Autodesk Fusion 360 part; units mm, degrees
(part 2 of 2)
  spline S13 degree 5 poles (-231.6326, -210.6007) (-231.5801, -210.5749) (-231.4751, -210.5231) (-231.318, -210.4449) (-231.1091, -210.34) (-230.8492, -210.2076) (-230.5904, -210.0739) (-230.3328, -209.9389) (-230.0763, -209.8027) (-229.821, -209.6652) (-229.5668, -209.5264) (-229.3139, -209.3863) (-229.0621, -209.245) (-228.8116, -209.1023) (-228.5623, -208.9584) (-228.3143, -208.8132) (-228.0675, -208.6668) (-227.8221, -208.5191) (-227.5779, -208.37) (-227.335, -208.2197) (-227.0934, -208.0681) (-226.8532, -207.9153) (-226.6143, -207.7611) (-226.3769, -207.6057) (-226.1408, -207.4489) (-225.9061, -207.2909) (-225.6728, -207.1316) (-225.4409, -206.971) (-225.2106, -206.8091) (-224.9817, -206.6459) (-224.7543, -206.4813) (-224.5284, -206.3155) (-224.304, -206.1484) (-224.0813, -205.9799) (-223.8601, -205.8102) (-223.6405, -205.6391) (-223.4226, -205.4667) (-223.2062, -205.2929) (-222.9916, -205.1179) (-222.7786, -204.9415) (-222.5674, -204.7638) (-222.358, -204.5847) (-222.1504, -204.4042) (-221.9447, -204.2224) (-221.7408, -204.0391) (-221.5388, -203.8546) (-221.3387, -203.6686) (-221.1405, -203.4813) (-220.9443, -203.2926) (-220.75, -203.1025) (-220.5579, -202.911) (-220.368, -202.718) (-220.1805, -202.5234) (-219.9954, -202.3273) (-219.8127, -202.1296) (-219.6323, -201.9304) (-219.4541, -201.7299) (-219.278, -201.528) (-219.104, -201.3248) (-218.9326, -201.12) (-218.7643, -200.9135) (-218.5996, -200.7049) (-218.4389, -200.494) (-218.2823, -200.2809) (-218.1292, -200.0659) (-217.979, -199.8493) (-217.8307, -199.6317) (-217.6843, -199.4131) (-217.5406, -199.1931) (-217.4019, -198.9707) (-217.2716, -198.7443) (-217.1767, -198.5586) (-217.112, -198.4162) (-217.0719, -198.3197) (-217.0526, -198.2711) knots -1 -1 -1 -1 -1 -1 -0.98571429 -0.97142857 -0.95714286 -0.94285714 -0.92857143 -0.91428571 -0.9 -0.88571429 -0.87142857 -0.85714286 -0.84285714 -0.82857143 -0.81428571 -0.8 -0.78571429 -0.77142857 -0.75714286 -0.74285714 -0.72857143 -0.71428571 -0.7 -0.68571429 -0.67142857 -0.65714286 -0.64285714 -0.62857143 -0.61428571 -0.6 -0.58571429 -0.57142857 -0.55714286 -0.54285714 -0.52857143 -0.51428571 -0.5 -0.48571429 -0.47142857 -0.45714286 -0.44285714 -0.42857143 -0.41428571 -0.4 -0.38571429 -0.37142857 -0.35714286 -0.34285714 -0.32857143 -0.31428571 -0.3 -0.28571429 -0.27142857 -0.25714286 -0.24285714 -0.22857143 -0.21428571 -0.2 -0.18571429 -0.17142857 -0.15714286 -0.14285714 -0.12857143 -0.11428571 -0.1 -0.08571429 -0.07142857 -0.05714286 -0.04285714 -0.02857143 -0.01428571 0 0 0 0 0 0
  line L13 (-217.0526, -198.2711) -> (-214.0537, -190.7145)
  arc A27 (-211.5159, -189.5709) -> (-214.0537, -190.7145) centre (-212.1947, -191.4522) ccw
  arc A28 (-211.5159, -189.5709) -> (-201.4878, -192.2579) centre (-190.6397, -131.7161) ccw
  arc A29 (-199.8618, -194.5172) -> (-201.4878, -192.2579) centre (-201.8406, -194.2266) ccw
  line L14 (-199.8618, -194.5172) -> (-201.043, -202.5609)
  spline S14 degree 5 poles (-201.043, -202.5609) (-201.0506, -202.6126) (-201.0641, -202.7162) (-201.0793, -202.8719) (-201.09, -203.0801) (-201.0903, -203.3414) (-201.0814, -203.6034) (-201.0669, -203.8657) (-201.0494, -204.1282) (-201.0299, -204.3908) (-201.008, -204.6535) (-200.983, -204.9163) (-200.9539, -205.1791) (-200.9201, -205.4421) (-200.8818, -205.7051) (-200.8393, -205.9681) (-200.7932, -206.2312) (-200.7443, -206.4941) (-200.6927, -206.757) (-200.6386, -207.0198) (-200.5819, -207.2825) (-200.5225, -207.545) (-200.4603, -207.8074) (-200.3952, -208.0696) (-200.3273, -208.3318) (-200.2567, -208.5937) (-200.1835, -208.8554) (-200.1078, -209.117) (-200.0298, -209.3783) (-199.9495, -209.6394) (-199.8669, -209.9002) (-199.782, -210.1609) (-199.6947, -210.4212) (-199.6052, -210.6813) (-199.5133, -210.9411) (-199.4193, -211.2006) (-199.3231, -211.4598) (-199.2247, -211.7188) (-199.1242, -211.9774) (-199.0217, -212.2357) (-198.9171, -212.4936) (-198.8104, -212.7512) (-198.7017, -213.0085) (-198.591, -213.2654) (-198.4783, -213.522) (-198.3636, -213.7781) (-198.247, -214.0339) (-198.1284, -214.2893) (-198.008, -214.5444) (-197.8856, -214.799) (-197.7613, -215.0532) (-197.6352, -215.307) (-197.5073, -215.5603) (-197.3775, -215.8133) (-197.2459, -216.0658) (-197.1125, -216.3178) (-196.9773, -216.5694) (-196.8403, -216.8206) (-196.7016, -217.0713) (-196.5611, -217.3215) (-196.4189, -217.5712) (-196.275, -217.8205) (-196.1294, -218.0693) (-195.982, -218.3175) (-195.833, -218.5653) (-195.6823, -218.8126) (-195.53, -219.0593) (-195.376, -219.3056) (-195.2203, -219.5513) (-195.063, -219.7965) (-194.9042, -220.0411) (-194.7758, -220.2364) (-194.6787, -220.3826) (-194.6137, -220.48) (-194.5811, -220.5287) knots 0 0 0 0 0 0 0.01428571 0.02857143 0.04285714 0.05714286 0.07142857 0.08571429 0.1 0.11428571 0.12857143 0.14285714 0.15714286 0.17142857 0.18571429 0.2 0.21428571 0.22857143 0.24285714 0.25714286 0.27142857 0.28571429 0.3 0.31428571 0.32857143 0.34285714 0.35714286 0.37142857 0.38571429 0.4 0.41428571 0.42857143 0.44285714 0.45714286 0.47142857 0.48571429 0.5 0.51428571 0.52857143 0.54285714 0.55714286 0.57142857 0.58571429 0.6 0.61428571 0.62857143 0.64285714 0.65714286 0.67142857 0.68571429 0.7 0.71428571 0.72857143 0.74285714 0.75714286 0.77142857 0.78571429 0.8 0.81428571 0.82857143 0.84285714 0.85714286 0.87142857 0.88571429 0.9 0.91428571 0.92857143 0.94285714 0.95714286 0.97142857 0.98571429 1 1 1 1 1 1
  arc A30 (-194.5811, -220.5287) -> (-186.6983, -220.5287) centre (-190.6397, -131.7161) ccw
  spline S15 degree 5 poles (-186.6983, -220.5287) (-186.6657, -220.48) (-186.6007, -220.3826) (-186.5037, -220.2364) (-186.3753, -220.0411) (-186.2164, -219.7965) (-186.0591, -219.5513) (-185.9035, -219.3056) (-185.7495, -219.0593) (-185.5971, -218.8126) (-185.4464, -218.5653) (-185.2974, -218.3175) (-185.1501, -218.0693) (-185.0044, -217.8205) (-184.8605, -217.5712) (-184.7183, -217.3215) (-184.5778, -217.0713) (-184.4391, -216.8206) (-184.3021, -216.5694) (-184.1669, -216.3178) (-184.0335, -216.0658) (-183.9019, -215.8133) (-183.7721, -215.5603) (-183.6442, -215.307) (-183.5181, -215.0532) (-183.3938, -214.799) (-183.2715, -214.5444) (-183.151, -214.2893) (-183.0324, -214.0339) (-182.9158, -213.7781) (-182.8011, -213.522) (-182.6884, -213.2654) (-182.5777, -213.0085) (-182.469, -212.7512) (-182.3624, -212.4936) (-182.2577, -212.2357) (-182.1552, -211.9774) (-182.0547, -211.7188) (-181.9564, -211.4598) (-181.8601, -211.2006) (-181.7661, -210.9411) (-181.6743, -210.6813) (-181.5847, -210.4212) (-181.4975, -210.1609) (-181.4125, -209.9002) (-181.3299, -209.6394) (-181.2496, -209.3783) (-181.1716, -209.117) (-181.096, -208.8554) (-181.0228, -208.5937) (-180.9521, -208.3318) (-180.8842, -208.0696) (-180.8191, -207.8074) (-180.7569, -207.545) (-180.6975, -207.2825) (-180.6409, -207.0198) (-180.5868, -206.757) (-180.5352, -206.4941) (-180.4862, -206.2312) (-180.4401, -205.9681) (-180.3976, -205.7051) (-180.3593, -205.4421) (-180.3255, -205.1791) (-180.2964, -204.9163) (-180.2714, -204.6535) (-180.2496, -204.3908) (-180.23, -204.1282) (-180.2125, -203.8657) (-180.1981, -203.6034) (-180.1891, -203.3414) (-180.1895, -203.0801) (-180.2001, -202.8719) (-180.2153, -202.7162) (-180.2288, -202.6126) (-180.2364, -202.5609) knots -1 -1 -1 -1 -1 -1 -0.98571429 -0.97142857 -0.95714286 -0.94285714 -0.92857143 -0.91428571 -0.9 -0.88571429 -0.87142857 -0.85714286 -0.84285714 -0.82857143 -0.81428571 -0.8 -0.78571429 -0.77142857 -0.75714286 -0.74285714 -0.72857143 -0.71428571 -0.7 -0.68571429 -0.67142857 -0.65714286 -0.64285714 -0.62857143 -0.61428571 -0.6 -0.58571429 -0.57142857 -0.55714286 -0.54285714 -0.52857143 -0.51428571 -0.5 -0.48571429 -0.47142857 -0.45714286 -0.44285714 -0.42857143 -0.41428571 -0.4 -0.38571429 -0.37142857 -0.35714286 -0.34285714 -0.32857143 -0.31428571 -0.3 -0.28571429 -0.27142857 -0.25714286 -0.24285714 -0.22857143 -0.21428571 -0.2 -0.18571429 -0.17142857 -0.15714286 -0.14285714 -0.12857143 -0.11428571 -0.1 -0.08571429 -0.07142857 -0.05714286 -0.04285714 -0.02857143 -0.01428571 0 0 0 0 0 0
  line L15 (-180.2364, -202.5609) -> (-181.4176, -194.5172)
  arc A31 (-179.7916, -192.2579) -> (-181.4176, -194.5172) centre (-179.4388, -194.2266) ccw
  arc A32 (-179.7916, -192.2579) -> (-169.7635, -189.5709) centre (-190.6397, -131.7161) ccw
  arc A33 (-167.2257, -190.7145) -> (-169.7635, -189.5709) centre (-169.0847, -191.4522) ccw
  line L16 (-167.2257, -190.7145) -> (-164.2268, -198.2711)
  spline S16 degree 5 poles (-164.2268, -198.2711) (-164.2075, -198.3197) (-164.1675, -198.4162) (-164.1028, -198.5586) (-164.0079, -198.7443) (-163.8775, -198.9707) (-163.7388, -199.1931) (-163.5951, -199.4131) (-163.4487, -199.6317) (-163.3005, -199.8493) (-163.1502, -200.0659) (-162.9972, -200.2809) (-162.8405, -200.494) (-162.6798, -200.7049) (-162.5151, -200.9135) (-162.3468, -201.12) (-162.1754, -201.3248) (-162.0015, -201.528) (-161.8253, -201.7299) (-161.6471, -201.9304) (-161.4667, -202.1296) (-161.284, -202.3273) (-161.099, -202.5234) (-160.9114, -202.718) (-160.7216, -202.911) (-160.5294, -203.1025) (-160.3352, -203.2926) (-160.1389, -203.4813) (-159.9407, -203.6686) (-159.7406, -203.8546) (-159.5386, -204.0391) (-159.3348, -204.2224) (-159.129, -204.4042) (-158.9214, -204.5847) (-158.712, -204.7638) (-158.5008, -204.9415) (-158.2878, -205.1179) (-158.0732, -205.2929) (-157.8569, -205.4667) (-157.6389, -205.6391) (-157.4193, -205.8102) (-157.1982, -205.9799) (-156.9754, -206.1484) (-156.7511, -206.3155) (-156.5252, -206.4813) (-156.2978, -206.6459) (-156.0689, -206.8091) (-155.8385, -206.971) (-155.6067, -207.1316) (-155.3734, -207.2909) (-155.1387, -207.4489) (-154.9026, -207.6057) (-154.6651, -207.7611) (-154.4262, -207.9153) (-154.186, -208.0681) (-153.9444, -208.2197) (-153.7016, -208.37) (-153.4574, -208.5191) (-153.2119, -208.6668) (-152.9651, -208.8132) (-152.7171, -208.9584) (-152.4678, -209.1023) (-152.2173, -209.245) (-151.9656, -209.3863) (-151.7126, -209.5264) (-151.4585, -209.6652) (-151.2031, -209.8027) (-150.9467, -209.9389) (-150.689, -210.0739) (-150.4302, -210.2076) (-150.1703, -210.34) (-149.9615, -210.4449) (-149.8043, -210.5231) (-149.6993, -210.5749) (-149.6468, -210.6007) knots 0 0 0 0 0 0 0.01428571 0.02857143 0.04285714 0.05714286 0.07142857 0.08571429 0.1 0.11428571 0.12857143 0.14285714 0.15714286 0.17142857 0.18571429 0.2 0.21428571 0.22857143 0.24285714 0.25714286 0.27142857 0.28571429 0.3 0.31428571 0.32857143 0.34285714 0.35714286 0.37142857 0.38571429 0.4 0.41428571 0.42857143 0.44285714 0.45714286 0.47142857 0.48571429 0.5 0.51428571 0.52857143 0.54285714 0.55714286 0.57142857 0.58571429 0.6 0.61428571 0.62857143 0.64285714 0.65714286 0.67142857 0.68571429 0.7 0.71428571 0.72857143 0.74285714 0.75714286 0.77142857 0.78571429 0.8 0.81428571 0.82857143 0.84285714 0.85714286 0.87142857 0.88571429 0.9 0.91428571 0.92857143 0.94285714 0.95714286 0.97142857 0.98571429 1 1 1 1 1 1
  arc A34 (-149.6468, -210.6007) -> (-142.8201, -206.6593) centre (-190.6397, -131.7161) ccw
  spline S17 degree 5 poles (-142.8201, -206.6593) (-142.8162, -206.6009) (-142.8086, -206.484) (-142.7976, -206.3089) (-142.7841, -206.0756) (-142.7688, -205.7843) (-142.7552, -205.4933) (-142.7433, -205.2027) (-142.733, -204.9124) (-142.7244, -204.6226) (-142.7176, -204.3331) (-142.7124, -204.044) (-142.7089, -203.7553) (-142.7072, -203.467) (-142.7072, -203.1792) (-142.7089, -202.8918) (-142.7124, -202.6049) (-142.7176, -202.3184) (-142.7245, -202.0324) (-142.7332, -201.7469) (-142.7437, -201.462) (-142.756, -201.1775) (-142.7701, -200.8935) (-142.786, -200.6101) (-142.8036, -200.3273) (-142.8232, -200.045) (-142.8445, -199.7633) (-142.8677, -199.4823) (-142.8927, -199.2018) (-142.9196, -198.922) (-142.9484, -198.6428) (-142.979, -198.3642) (-143.0116, -198.0864) (-143.0461, -197.8092) (-143.0825, -197.5328) (-143.1209, -197.2571) (-143.1612, -196.9821) (-143.2035, -196.7079) (-143.2478, -196.4345) (-143.2941, -196.1619) (-143.3424, -195.8901) (-143.3928, -195.6192) (-143.4453, -195.3492) (-143.4999, -195.0801) (-143.5566, -194.812) (-143.6155, -194.5447) (-143.6765, -194.2785) (-143.7396, -194.0132) (-143.8049, -193.7488) (-143.8724, -193.4856) (-143.9422, -193.2234) (-144.0144, -192.9625) (-144.0892, -192.7028) (-144.1665, -192.4444) (-144.2463, -192.1874) (-144.3286, -191.9316) (-144.4131, -191.677) (-144.4999, -191.4235) (-144.589, -191.1713) (-144.6806, -190.9204) (-144.7753, -190.6714) (-144.8736, -190.4244) (-144.9759, -190.1798) (-145.0821, -189.9377) (-145.1918, -189.6976) (-145.3042, -189.4592) (-145.4186, -189.222) (-145.5347, -188.9859) (-145.6533, -188.7515) (-145.7766, -188.5202) (-145.9075, -188.2941) (-146.0209, -188.119) (-146.1119, -187.9918) (-146.1754, -187.9088) (-146.2078, -187.8678) knots -1 -1 -1 -1 -1 -1 -0.98571429 -0.97142857 -0.95714286 -0.94285714 -0.92857143 -0.91428571 -0.9 -0.88571429 -0.87142857 -0.85714286 -0.84285714 -0.82857143 -0.81428571 -0.8 -0.78571429 -0.77142857 -0.75714286 -0.74285714 -0.72857143 -0.71428571 -0.7 -0.68571429 -0.67142857 -0.65714286 -0.64285714 -0.62857143 -0.61428571 -0.6 -0.58571429 -0.57142857 -0.55714286 -0.54285714 -0.52857143 -0.51428571 -0.5 -0.48571429 -0.47142857 -0.45714286 -0.44285714 -0.42857143 -0.41428571 -0.4 -0.38571429 -0.37142857 -0.35714286 -0.34285714 -0.32857143 -0.31428571 -0.3 -0.28571429 -0.27142857 -0.25714286 -0.24285714 -0.22857143 -0.21428571 -0.2 -0.18571429 -0.17142857 -0.15714286 -0.14285714 -0.12857143 -0.11428571 -0.1 -0.08571429 -0.07142857 -0.05714286 -0.04285714 -0.02857143 -0.01428571 0 0 0 0 0 0
  line L17 (-146.2078, -187.8678) -> (-151.2526, -181.4924)
  arc A35 (-150.974, -178.7228) -> (-151.2526, -181.4924) centre (-149.6842, -180.2513) ccw
  arc A36 (-150.974, -178.7228) -> (-143.633, -171.3818) centre (-190.6397, -131.7161) ccw
  arc A37 (-140.8634, -171.1032) -> (-143.633, -171.3818) centre (-142.1045, -172.6716) ccw
  line L18 (-140.8634, -171.1032) -> (-134.488, -176.148)
  spline S18 degree 5 poles (-134.488, -176.148) (-134.447, -176.1804) (-134.364, -176.2439) (-134.2368, -176.3349) (-134.0617, -176.4483) (-133.8356, -176.5792) (-133.6043, -176.7024) (-133.3699, -176.8211) (-133.1338, -176.9372) (-132.8966, -177.0516) (-132.6582, -177.164) (-132.4181, -177.2737) (-132.1759, -177.3799) (-131.9313, -177.4822) (-131.6844, -177.5805) (-131.4353, -177.6752) (-131.1845, -177.7668) (-130.9323, -177.8559) (-130.6788, -177.9427) (-130.4242, -178.0272) (-130.1684, -178.1095) (-129.9114, -178.1893) (-129.653, -178.2666) (-129.3933, -178.3414) (-129.1324, -178.4136) (-128.8702, -178.4834) (-128.6069, -178.5509) (-128.3426, -178.6161) (-128.0773, -178.6793) (-127.811, -178.7403) (-127.5438, -178.7991) (-127.2757, -178.8559) (-127.0066, -178.9105) (-126.7366, -178.963) (-126.4656, -179.0134) (-126.1939, -179.0617) (-125.9213, -179.108) (-125.6478, -179.1522) (-125.3736, -179.1945) (-125.0987, -179.2349) (-124.823, -179.2732) (-124.5466, -179.3097) (-124.2694, -179.3442) (-123.9916, -179.3768) (-123.713, -179.4074) (-123.4338, -179.4362) (-123.154, -179.4631) (-122.8735, -179.4881) (-122.5924, -179.5113) (-122.3108, -179.5326) (-122.0285, -179.5521) (-121.7456, -179.5698) (-121.4622, -179.5857) (-121.1783, -179.5998) (-120.8938, -179.6121) (-120.6088, -179.6225) (-120.3233, -179.6313) (-120.0374, -179.6382) (-119.7509, -179.6434) (-119.464, -179.6469) (-119.1766, -179.6486) (-118.8888, -179.6486) (-118.6005, -179.6468) (-118.3118, -179.6434) (-118.0227, -179.6382) (-117.7332, -179.6313) (-117.4433, -179.6228) (-117.1531, -179.6125) (-116.8625, -179.6006) (-116.5715, -179.587) (-116.2802, -179.5717) (-116.0469, -179.5581) (-115.8717, -179.5472) (-115.7549, -179.5396) (-115.6965, -179.5357) knots 0 0 0 0 0 0 0.01428571 0.02857143 0.04285714 0.05714286 0.07142857 0.08571429 0.1 0.11428571 0.12857143 0.14285714 0.15714286 0.17142857 0.18571429 0.2 0.21428571 0.22857143 0.24285714 0.25714286 0.27142857 0.28571429 0.3 0.31428571 0.32857143 0.34285714 0.35714286 0.37142857 0.38571429 0.4 0.41428571 0.42857143 0.44285714 0.45714286 0.47142857 0.48571429 0.5 0.51428571 0.52857143 0.54285714 0.55714286 0.57142857 0.58571429 0.6 0.61428571 0.62857143 0.64285714 0.65714286 0.67142857 0.68571429 0.7 0.71428571 0.72857143 0.74285714 0.75714286 0.77142857 0.78571429 0.8 0.81428571 0.82857143 0.84285714 0.85714286 0.87142857 0.88571429 0.9 0.91428571 0.92857143 0.94285714 0.95714286 0.97142857 0.98571429 1 1 1 1 1 1
  arc A38 (-115.6965, -179.5357) -> (-111.7551, -172.709) centre (-190.6397, -131.7161) ccw
  spline S19 degree 5 poles (-111.7551, -172.709) (-111.7809, -172.6564) (-111.8327, -172.5515) (-111.9109, -172.3943) (-112.0158, -172.1855) (-112.1482, -171.9255) (-112.2819, -171.6668) (-112.4169, -171.4091) (-112.5531, -171.1526) (-112.6906, -170.8973) (-112.8294, -170.6432) (-112.9695, -170.3902) (-113.1108, -170.1385) (-113.2535, -169.888) (-113.3974, -169.6387) (-113.5425, -169.3907) (-113.689, -169.1439) (-113.8367, -168.8984) (-113.9857, -168.6542) (-114.1361, -168.4113) (-114.2876, -168.1698) (-114.4405, -167.9296) (-114.5947, -167.6907) (-114.7501, -167.4532) (-114.9068, -167.2171) (-115.0649, -166.9824) (-115.2242, -166.7491) (-115.3848, -166.5173) (-115.5467, -166.2869) (-115.7099, -166.058) (-115.8744, -165.8306) (-116.0403, -165.6047) (-116.2074, -165.3804) (-116.3759, -165.1576) (-116.5456, -164.9364) (-116.7167, -164.7169) (-116.8891, -164.4989) (-117.0628, -164.2826) (-117.2379, -164.068) (-117.4143, -163.855) (-117.592, -163.6438) (-117.7711, -163.4344) (-117.9516, -163.2268) (-118.1334, -163.021) (-118.3166, -162.8172) (-118.5012, -162.6152) (-118.6872, -162.4151) (-118.8745, -162.2169) (-119.0632, -162.0206) (-119.2533, -161.8264) (-119.4448, -161.6342) (-119.6378, -161.4443) (-119.8324, -161.2568) (-120.0285, -161.0717) (-120.2262, -160.8891) (-120.4253, -160.7087) (-120.6259, -160.5304) (-120.8277, -160.3543) (-121.031, -160.1804) (-121.2358, -160.009) (-121.4423, -159.8407) (-121.6509, -159.676) (-121.8618, -159.5152) (-122.0748, -159.3586) (-122.2899, -159.2056) (-122.5064, -159.0553) (-122.7241, -158.9071) (-122.9427, -158.7607) (-123.1627, -158.617) (-123.3851, -158.4783) (-123.6115, -158.3479) (-123.7972, -158.253) (-123.9396, -158.1883) (-124.0361, -158.1482) (-124.0847, -158.129) knots -1 -1 -1 -1 -1 -1 -0.98571429 -0.97142857 -0.95714286 -0.94285714 -0.92857143 -0.91428571 -0.9 -0.88571429 -0.87142857 -0.85714286 -0.84285714 -0.82857143 -0.81428571 -0.8 -0.78571429 -0.77142857 -0.75714286 -0.74285714 -0.72857143 -0.71428571 -0.7 -0.68571429 -0.67142857 -0.65714286 -0.64285714 -0.62857143 -0.61428571 -0.6 -0.58571429 -0.57142857 -0.55714286 -0.54285714 -0.52857143 -0.51428571 -0.5 -0.48571429 -0.47142857 -0.45714286 -0.44285714 -0.42857143 -0.41428571 -0.4 -0.38571429 -0.37142857 -0.35714286 -0.34285714 -0.32857143 -0.31428571 -0.3 -0.28571429 -0.27142857 -0.25714286 -0.24285714 -0.22857143 -0.21428571 -0.2 -0.18571429 -0.17142857 -0.15714286 -0.14285714 -0.12857143 -0.11428571 -0.1 -0.08571429 -0.07142857 -0.05714286 -0.04285714 -0.02857143 -0.01428571 0 0 0 0 0 0
  line L19 (-124.0847, -158.129) -> (-131.6413, -155.13)
  arc A39 (-132.7849, -152.5923) -> (-131.6413, -155.13) centre (-130.9036, -153.2711) ccw
  arc A40 (-132.7849, -152.5923) -> (-130.0978, -142.5642) centre (-190.6397, -131.7161) ccw
  arc A41 (-127.8386, -140.9382) -> (-130.0978, -142.5642) centre (-128.1292, -142.9169) ccw
  line L20 (-127.8386, -140.9382) -> (-119.7949, -142.1194)
  spline S20 degree 5 poles (-119.7949, -142.1194) (-119.7432, -142.127) (-119.6396, -142.1405) (-119.4839, -142.1557) (-119.2756, -142.1663) (-119.0144, -142.1666) (-118.7524, -142.1577) (-118.4901, -142.1432) (-118.2276, -142.1258) (-117.9649, -142.1062) (-117.7023, -142.0844) (-117.4395, -142.0594) (-117.1767, -142.0303) (-116.9137, -141.9965) (-116.6507, -141.9581) (-116.3877, -141.9156) (-116.1246, -141.8696) (-115.8616, -141.8206) (-115.5988, -141.769) (-115.336, -141.7149) (-115.0733, -141.6583) (-114.8108, -141.5989) (-114.5484, -141.5367) (-114.2861, -141.4716) (-114.024, -141.4036) (-113.7621, -141.333) (-113.5004, -141.2598) (-113.2388, -141.1842) (-112.9775, -141.1062) (-112.7164, -141.0259) (-112.4555, -140.9433) (-112.1949, -140.8583) (-111.9346, -140.7711) (-111.6745, -140.6815) (-111.4147, -140.5897) (-111.1552, -140.4957) (-110.8959, -140.3994) (-110.637, -140.3011) (-110.3784, -140.2006) (-110.1201, -140.098) (-109.8622, -139.9934) (-109.6046, -139.8868) (-109.3473, -139.7781) (-109.0904, -139.6674) (-108.8338, -139.5546) (-108.5777, -139.44) (-108.3219, -139.3233) (-108.0664, -139.2048) (-107.8114, -139.0843) (-107.5568, -138.9619) (-107.3026, -138.8377) (-107.0488, -138.7116) (-106.7955, -138.5836) (-106.5425, -138.4539) (-106.29, -138.3223) (-106.038, -138.1889) (-105.7864, -138.0537) (-105.5352, -137.9167) (-105.2845, -137.778) (-105.0343, -137.6375) (-104.7846, -137.4953) (-104.5353, -137.3514) (-104.2865, -137.2057) (-104.0382, -137.0584) (-103.7905, -136.9094) (-103.5432, -136.7587) (-103.2964, -136.6063) (-103.0502, -136.4523) (-102.8045, -136.2967) (-102.5593, -136.1394) (-102.3147, -135.9805) (-102.1194, -135.8521) (-101.9732, -135.7551) (-101.8758, -135.6901) (-101.8271, -135.6575) knots 0 0 0 0 0 0 0.01428571 0.02857143 0.04285714 0.05714286 0.07142857 0.08571429 0.1 0.11428571 0.12857143 0.14285714 0.15714286 0.17142857 0.18571429 0.2 0.21428571 0.22857143 0.24285714 0.25714286 0.27142857 0.28571429 0.3 0.31428571 0.32857143 0.34285714 0.35714286 0.37142857 0.38571429 0.4 0.41428571 0.42857143 0.44285714 0.45714286 0.47142857 0.48571429 0.5 0.51428571 0.52857143 0.54285714 0.55714286 0.57142857 0.58571429 0.6 0.61428571 0.62857143 0.64285714 0.65714286 0.67142857 0.68571429 0.7 0.71428571 0.72857143 0.74285714 0.75714286 0.77142857 0.78571429 0.8 0.81428571 0.82857143 0.84285714 0.85714286 0.87142857 0.88571429 0.9 0.91428571 0.92857143 0.94285714 0.95714286 0.97142857 0.98571429 1 1 1 1 1 1
  arc A42 (-101.8271, -135.6575) -> (-101.8271, -127.7747) centre (-190.6397, -131.7161) ccw
  spline S21 degree 5 poles (-101.8271, -127.7747) (-101.8758, -127.7421) (-101.9732, -127.6771) (-102.1194, -127.58) (-102.3147, -127.4516) (-102.5593, -127.2927) (-102.8045, -127.1355) (-103.0502, -126.9798) (-103.2964, -126.8258) (-103.5432, -126.6735) (-103.7905, -126.5228) (-104.0382, -126.3738) (-104.2865, -126.2264) (-104.5353, -126.0808) (-104.7846, -125.9368) (-105.0343, -125.7946) (-105.2845, -125.6542) (-105.5352, -125.5154) (-105.7864, -125.3785) (-106.038, -125.2433) (-106.29, -125.1099) (-106.5425, -124.9783) (-106.7955, -124.8485) (-107.0488, -124.7205) (-107.3026, -124.5944) (-107.5568, -124.4702) (-107.8114, -124.3478) (-108.0664, -124.2274) (-108.3219, -124.1088) (-108.5777, -123.9922) (-108.8338, -123.8775) (-109.0904, -123.7648) (-109.3473, -123.6541) (-109.6046, -123.5454) (-109.8622, -123.4387) (-110.1201, -123.3341) (-110.3784, -123.2315) (-110.637, -123.1311) (-110.8959, -123.0327) (-111.1552, -122.9365) (-111.4147, -122.8424) (-111.6745, -122.7506) (-111.9346, -122.6611) (-112.1949, -122.5738) (-112.4555, -122.4889) (-112.7164, -122.4063) (-112.9775, -122.3259) (-113.2388, -122.248) (-113.5004, -122.1723) (-113.7621, -122.0991) (-114.024, -122.0285) (-114.2861, -121.9606) (-114.5484, -121.8955) (-114.8108, -121.8332) (-115.0733, -121.7739) (-115.336, -121.7172) (-115.5988, -121.6631) (-115.8616, -121.6115) (-116.1246, -121.5625) (-116.3877, -121.5165) (-116.6507, -121.474) (-116.9137, -121.4356) (-117.1767, -121.4019) (-117.4395, -121.3728) (-117.7023, -121.3478) (-117.9649, -121.3259) (-118.2276, -121.3064) (-118.4901, -121.2889) (-118.7524, -121.2744) (-119.0144, -121.2655) (-119.2756, -121.2658) (-119.4839, -121.2765) (-119.6396, -121.2917) (-119.7432, -121.3052) (-119.7949, -121.3128) knots -1 -1 -1 -1 -1 -1 -0.98571429 -0.97142857 -0.95714286 -0.94285714 -0.92857143 -0.91428571 -0.9 -0.88571429 -0.87142857 -0.85714286 -0.84285714 -0.82857143 -0.81428571 -0.8 -0.78571429 -0.77142857 -0.75714286 -0.74285714 -0.72857143 -0.71428571 -0.7 -0.68571429 -0.67142857 -0.65714286 -0.64285714 -0.62857143 -0.61428571 -0.6 -0.58571429 -0.57142857 -0.55714286 -0.54285714 -0.52857143 -0.51428571 -0.5 -0.48571429 -0.47142857 -0.45714286 -0.44285714 -0.42857143 -0.41428571 -0.4 -0.38571429 -0.37142857 -0.35714286 -0.34285714 -0.32857143 -0.31428571 -0.3 -0.28571429 -0.27142857 -0.25714286 -0.24285714 -0.22857143 -0.21428571 -0.2 -0.18571429 -0.17142857 -0.15714286 -0.14285714 -0.12857143 -0.11428571 -0.1 -0.08571429 -0.07142857 -0.05714286 -0.04285714 -0.02857143 -0.01428571 0 0 0 0 0 0
  line L21 (-119.7949, -121.3128) -> (-127.8386, -122.494)
  arc A43 (-130.0978, -120.8679) -> (-127.8386, -122.494) centre (-128.1292, -120.5152) ccw
  arc A44 (-130.0978, -120.8679) -> (-132.7849, -110.8399) centre (-190.6397, -131.7161) ccw
  arc A45 (-131.6413, -108.3021) -> (-132.7849, -110.8399) centre (-130.9036, -110.1611) ccw
  line L22 (-131.6413, -108.3021) -> (-124.0847, -105.3032)
  spline S22 degree 5 poles (-124.0847, -105.3032) (-124.0361, -105.2839) (-123.9396, -105.2438) (-123.7972, -105.1791) (-123.6115, -105.0842) (-123.3851, -104.9538) (-123.1627, -104.8152) (-122.9427, -104.6715) (-122.7241, -104.5251) (-122.5064, -104.3768) (-122.2899, -104.2265) (-122.0748, -104.0735) (-121.8618, -103.9169) (-121.6509, -103.7562) (-121.4423, -103.5915) (-121.2358, -103.4231) (-121.031, -103.2517) (-120.8277, -103.0778) (-120.6259, -102.9017) (-120.4253, -102.7235) (-120.2262, -102.5431) (-120.0285, -102.3604) (-119.8324, -102.1753) (-119.6378, -101.9878) (-119.4448, -101.7979) (-119.2533, -101.6058) (-119.0632, -101.4115) (-118.8745, -101.2152) (-118.6872, -101.017) (-118.5012, -100.8169) (-118.3166, -100.615) (-118.1334, -100.4111) (-117.9516, -100.2054) (-117.7711, -99.9978) (-117.592, -99.7883) (-117.4143, -99.5771) (-117.2379, -99.3642) (-117.0628, -99.1495) (-116.8891, -98.9332) (-116.7167, -98.7153) (-116.5456, -98.4957) (-116.3759, -98.2745) (-116.2074, -98.0518) (-116.0403, -97.8274) (-115.8744, -97.6015) (-115.7099, -97.3741) (-115.5467, -97.1452) (-115.3848, -96.9148) (-115.2242, -96.683) (-115.0649, -96.4497) (-114.9068, -96.215) (-114.7501, -95.9789) (-114.5947, -95.7414) (-114.4405, -95.5026) (-114.2876, -95.2624) (-114.1361, -95.0208) (-113.9857, -94.7779) (-113.8367, -94.5337) (-113.689, -94.2882) (-113.5425, -94.0415) (-113.3974, -93.7934) (-113.2535, -93.5442) (-113.1108, -93.2937) (-112.9695, -93.0419) (-112.8294, -92.789) (-112.6906, -92.5348) (-112.5531, -92.2795) (-112.4169, -92.023) (-112.2819, -91.7654) (-112.1482, -91.5066) (-112.0158, -91.2467) (-111.9109, -91.0378) (-111.8327, -90.8807) (-111.7809, -90.7757) (-111.7551, -90.7231) knots 0 0 0 0 0 0 0.01428571 0.02857143 0.04285714 0.05714286 0.07142857 0.08571429 0.1 0.11428571 0.12857143 0.14285714 0.15714286 0.17142857 0.18571429 0.2 0.21428571 0.22857143 0.24285714 0.25714286 0.27142857 0.28571429 0.3 0.31428571 0.32857143 0.34285714 0.35714286 0.37142857 0.38571429 0.4 0.41428571 0.42857143 0.44285714 0.45714286 0.47142857 0.48571429 0.5 0.51428571 0.52857143 0.54285714 0.55714286 0.57142857 0.58571429 0.6 0.61428571 0.62857143 0.64285714 0.65714286 0.67142857 0.68571429 0.7 0.71428571 0.72857143 0.74285714 0.75714286 0.77142857 0.78571429 0.8 0.81428571 0.82857143 0.84285714 0.85714286 0.87142857 0.88571429 0.9 0.91428571 0.92857143 0.94285714 0.95714286 0.97142857 0.98571429 1 1 1 1 1 1
  arc A46 (-111.7551, -90.7231) -> (-115.6965, -83.8964) centre (-190.6397, -131.7161) ccw
  spline S23 degree 5 poles (-115.6965, -83.8964) (-115.7549, -83.8925) (-115.8717, -83.8849) (-116.0469, -83.874) (-116.2802, -83.8604) (-116.5715, -83.8452) (-116.8625, -83.8315) (-117.1531, -83.8196) (-117.4433, -83.8094) (-117.7332, -83.8008) (-118.0227, -83.7939) (-118.3118, -83.7888) (-118.6005, -83.7853) (-118.8888, -83.7836) (-119.1766, -83.7835) (-119.464, -83.7853) (-119.7509, -83.7887) (-120.0374, -83.7939) (-120.3233, -83.8009) (-120.6088, -83.8096) (-120.8938, -83.8201) (-121.1783, -83.8324) (-121.4622, -83.8464) (-121.7456, -83.8623) (-122.0285, -83.88) (-122.3108, -83.8995) (-122.5924, -83.9208) (-122.8735, -83.944) (-123.154, -83.9691) (-123.4338, -83.9959) (-123.713, -84.0247) (-123.9916, -84.0554) (-124.2694, -84.088) (-124.5466, -84.1225) (-124.823, -84.1589) (-125.0987, -84.1973) (-125.3736, -84.2376) (-125.6478, -84.2799) (-125.9213, -84.3242) (-126.1939, -84.3705) (-126.4656, -84.4188) (-126.7366, -84.4692) (-127.0066, -84.5216) (-127.2757, -84.5763) (-127.5438, -84.633) (-127.811, -84.6919) (-128.0773, -84.7529) (-128.3426, -84.816) (-128.6069, -84.8813) (-128.8702, -84.9487) (-129.1324, -85.0185) (-129.3933, -85.0908) (-129.653, -85.1655) (-129.9114, -85.2428) (-130.1684, -85.3227) (-130.4242, -85.4049) (-130.6788, -85.4895) (-130.9323, -85.5762) (-131.1845, -85.6653) (-131.4353, -85.7569) (-131.6844, -85.8517) (-131.9313, -85.95) (-132.1759, -86.0522) (-132.4181, -86.1584) (-132.6582, -86.2681) (-132.8966, -86.3806) (-133.1338, -86.4949) (-133.3699, -86.6111) (-133.6043, -86.7297) (-133.8356, -86.8529) (-134.0617, -86.9839) (-134.2368, -87.0972) (-134.364, -87.1882) (-134.447, -87.2517) (-134.488, -87.2842) knots -1 -1 -1 -1 -1 -1 -0.98571429 -0.97142857 -0.95714286 -0.94285714 -0.92857143 -0.91428571 -0.9 -0.88571429 -0.87142857 -0.85714286 -0.84285714 -0.82857143 -0.81428571 -0.8 -0.78571429 -0.77142857 -0.75714286 -0.74285714 -0.72857143 -0.71428571 -0.7 -0.68571429 -0.67142857 -0.65714286 -0.64285714 -0.62857143 -0.61428571 -0.6 -0.58571429 -0.57142857 -0.55714286 -0.54285714 -0.52857143 -0.51428571 -0.5 -0.48571429 -0.47142857 -0.45714286 -0.44285714 -0.42857143 -0.41428571 -0.4 -0.38571429 -0.37142857 -0.35714286 -0.34285714 -0.32857143 -0.31428571 -0.3 -0.28571429 -0.27142857 -0.25714286 -0.24285714 -0.22857143 -0.21428571 -0.2 -0.18571429 -0.17142857 -0.15714286 -0.14285714 -0.12857143 -0.11428571 -0.1 -0.08571429 -0.07142857 -0.05714286 -0.04285714 -0.02857143 -0.01428571 0 0 0 0 0 0
  line L23 (-134.488, -87.2842) -> (-140.8634, -92.3289)
  arc A47 (-143.633, -92.0504) -> (-140.8634, -92.3289) centre (-142.1045, -90.7606) ccw
  circle A48 centre (-190.6397, -131.7161) radius 5
  circle A49 centre (-190.6397, -131.7161) radius 5
  dimension "d22" = 10
  constraint concentric A0 A49
  measures "d22" diameter of A49
copy_body "Body->Comp1" bodies 2 removing the originals makes body 3 in component "Component"
extrude "Extrude1''" add sketch "Sketch2" along normal blind 20 and the other way blind 31.7 contours A48 A49 sketch seen with x (-0.5, 0.866025, 0) y (-0.866025, -0.5, 0) z (0, 0, 1) at (209.3893, -99.2408, 2.1005) bodies 3 in component "Component"
component "Spur Gear 12 teeth" placed x (-0.5, -0.866025, 0) y (0.866025, -0.5, 0) z (0, 0, 1) at (195.1331, 140.6804, -23.0796)
component "Spur Gear 24 teeth" placed x (1, 0, 0) y (0, 1, 0) z (0, 0, 1) at (0, 0, -23.8005)
component "Component" placed x (1, 0, 0) y (0, 1, 0) z (0, 0, 1) at (0, 0, -30) in component "Spur Gear 12 teeth"
